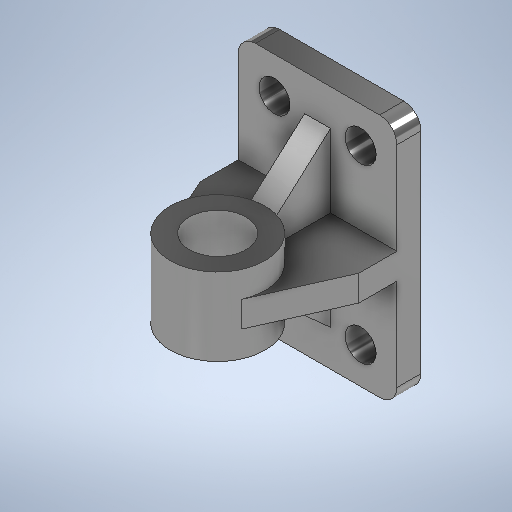
# Autodesk Inventor part: cad@55
Saved by Autodesk Inventor 2025.2 (Build 292293000, 293)
## iProperties
Created: 2025-04-10
Part Number: cad@55
Material: Generic
Document SubType Name: Modeling
Designer: spars
Density: 1 g/cm^3
Appearance: Chrome - Polished Black
Author: spars
Autodesk Inventor part; units mm, degrees
ref_plane "YZ Plane" through (0, 0, 0) normal (1, 0, 0) x (0, 1, 0)
ref_plane "XZ Plane" through (0, 0, 0) normal (0, 1, 0) x (-1, 0, 0)
ref_plane "XY Plane" through (0, 0, 0) normal (0, 0, 1) x (1, 0, 0)
sketch "Sketch1" plane through (0, 0, 0) normal (0, 0, 1) x (1, 0, 0)
  line L0 (-485.8468, 29.4924) -> (-321.1558, 29.4924) construction
  line L1 (-321.1558, 29.4924) -> (-321.1558, -92.2265) construction
  line L2 (-321.1558, -92.2265) -> (-485.8468, -92.2265) construction
  line L3 (-485.8468, -92.2265) -> (-485.8468, 29.4924) construction
  line L4 (-36, 71) -> (36, 71)
  line L5 (46, 61) -> (46, -61)
  line L6 (36, -71) -> (-36, -71)
  line L7 (-46, -61) -> (-46, 61)
  circle A0 centre (25, -50) radius 9
  circle A1 centre (-25, -50) radius 9
  circle A2 centre (25, 50) radius 9
  circle A3 centre (-25, 50) radius 9
  arc A4 (46, 61) -> (36, 71) centre (36, 61) ccw
  arc A5 (-46, -61) -> (-36, -71) centre (-36, -61) ccw
  arc A6 (-36, 71) -> (-46, 61) centre (-36, 61) ccw
  arc A7 (36, -71) -> (46, -61) centre (36, -61) ccw
  point P0 (0, 0)
  dimension "d9" = 18
  dimension "d15" = 50
  dimension "d18" = 100
  dimension "d23" = 10
  dimension "d24" = 10
  dimension "d25" = 10
  dimension "d26" = 21
  dimension "d27" = 21
  constraints: 8 centre point, 8 end point, 8 point on circle, 8 tangent, 2 horizontal, 2 parallel, 1 equal radius, 1 perpendicular, 1 vertical, 8 other
  measures "d9" diameter of A0
  measures "d15" distance of A0.centre A1.centre
  measures "d18" distance of A0.centre A2.centre
  measures "d23" radius of A4
  measures "d24" radius of A5
  measures "d25" radius of A7
  measures "d26" distance from line of L6 A0.centre
  measures "d27" distance from line of A2.centre L4
extrude "Extrusion1" add sketch "Sketch1" along normal blind 14
sketch "Sketch2" plane through (0, 0, 0) normal (0, 1, 0) x (-1, 0, 0)
  line L0 (-36, 14) -> (36, 14) projected
  point P0 (0, 0)
extrude "Extrusion2" [suppressed]
sketch "Sketch3" plane through (0, 0, 0) normal (0, 1, 0) x (-1, 0, 0)
  line L0 (-46, 0) -> (-46, 14) projected
  circle A0 centre (0, 72) radius 27.5 projected
  point P0 (0, 0)
sketch "Sketch4" plane through (0, 0, 0) normal (0, 1, 0) x (-1, 0, 0)
  line L0 (0, 72) -> (-9.6355, 72)
  line L1 (36, 14) -> (-36, 14) projected
  arc A0 (-25.1483, 83.127) -> (25.1483, 83.127) centre (0, 72) ccw
  line L2 (46, 0) -> (46, 14) projected
  line L3 (46, 14) -> (46, 36)
  line L4 (46, 36) -> (25.1483, 83.127)
  line L5 (-36, 14) -> (-46, 14) projected
  line L6 (-46, 14) -> (-46, 36)
  line L7 (-46, 36) -> (-25.1483, 83.127)
  line L8 (46, 14) -> (-46, 14)
  point P0 (0, 0)
  dimension "d36" = 58
  dimension "d37" = 55
  dimension "d38" = 22
  dimension "d39" = 22
  constraints: 12 end point, 2 point on circle, 2 tangent, 2 vertical, 1 centre point, 1 coincident, 1 horizontal, 1 perpendicular
  measures "d36" distance between parallel lines of L1 L0
  measures "d37" diameter of A0
  measures "d38" distance of L2.end L3.end
  measures "d39" distance of L5.end L6.end
extrude "Extrusion3" add sketch "Sketch4" along normal mid plane 15
sketch "Sketch5" plane through (0, 0, 0) normal (0, 1, 0) x (-1, 0, 0)
  arc A0 (-25.1483, 83.127) -> (25.1483, 83.127) centre (0, 72) ccw projected
  circle A1 centre (0, 72) radius 27.5
  circle A2 centre (0, 72) radius 16.5
  point P0 (0, 0)
  point P1 (25.1483, 83.127)
  point P2 (-25.1483, 83.127)
  dimension "d42" = 55
  dimension "d43" = 33
  constraints: 2 centre point, 2 coincident
  measures "d42" diameter of A1
  measures "d43" diameter of A2
extrude "Extrusion4" add sketch "Sketch5" along normal mid plane 45
sketch "Sketch6" plane through (0, 0, 0) normal (1, 0, 0) x (0, 1, 0)
  point P0 (0, 0)
sketch "Sketch7" plane through (0, 0, 14) normal (0, 0, 1) x (1, 0, 0)
  circle A0 centre (-25, -50) radius 9 projected
  circle A1 centre (25, -50) radius 9 projected
  line L0 (-25, -50) -> (25, -50)
  line L1 (0, -61.7432) -> (0, -41)
  point P0 (0, 0)
  constraints: 4 end point, 1 horizontal, 1 vertical
sketch "Sketch8" plane through (0, 0, 0) normal (1, 0, 0) x (0, 1, 0)
  point P0 (0, 0)
sketch "Sketch9" plane through (0, 0, 0) normal (1, 0, 0) x (0, 1, 0)
  line L0 (-41.1062, 23.8802) -> (-28.1794, 38.255)
  point P0 (0, 0)
  constraints: 2 end point
extrude "Rib1" add sketch "Sketch9" along normal mid plane 15 rib yes fills toward (-34.6057, 31.0342) open curves L0
ref_plane "Work Plane1" through (0, 0, 0) normal (0, -1, 0) x (1, 0, 0)
mirror "Mirror1" about plane through (0, 0, 0) normal (0, -1, 0) of "Rib1"
body "Solid1"
